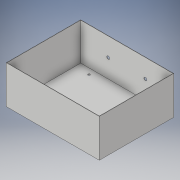
# Autodesk Inventor part: 563-AC-1404-4xSplitter
Saved by Autodesk Inventor 2018 (Build 220112000, 112)
## iProperties
Created: 2018-04-30
Part Number: 563-AC-1404-4xSplitter
Material: Generic
Document SubType Name: Modeling
Designer: bbramman
Density: 1 g/cm^3
Appearance: Default
Author: bbramman
Autodesk Inventor part; units mm, degrees
ref_plane "YZ Plane" through (0, 0, 0) normal (1, 0, 0) x (0, 1, 0)
ref_plane "XZ Plane" through (0, 0, 0) normal (0, 1, 0) x (-1, 0, 0)
ref_plane "XY Plane" through (0, 0, 0) normal (0, 0, 1) x (1, 0, 0)
sketch "Sketch1" plane through (0, 0, 0) normal (0, 1, 0) x (-1, 0, 0)
  line L0 (-63.5, 50.8) -> (63.5, 50.8)
  line L1 (63.5, 50.8) -> (63.5, -50.8)
  line L2 (63.5, -50.8) -> (-63.5, -50.8)
  line L3 (-63.5, -50.8) -> (-63.5, 50.8)
  line L4 (-63.5, 50.8) -> (63.5, -50.8) construction
  line L5 (63.5, 50.8) -> (-63.5, -50.8) construction
  point P0 (0, 0)
  dimension "d0" = 127
  dimension "d1" = 101.6
  constraints: 12 end point, 2 midpoint, 2 parallel, 1 horizontal, 1 perpendicular
  measures "d0" distance of L1.end L2.end
  measures "d1" distance of L0.end L1.end
extrude "Extrusion1" add sketch "Sketch1" along normal blind 1.016
sketch "Sketch2" plane through (0, 1.016, 0) normal (0, 1, 0) x (1, 0, 0)
  line L0 (63.5, 50.8) -> (-63.5, 50.8) projected
  line L1 (63.5, -50.8) -> (-63.5, -50.8)
  line L2 (-63.5, -50.8) -> (-63.5, 50.8)
  line L3 (-63.5, 50.8) -> (63.5, 50.8)
  line L4 (63.5, 50.8) -> (63.5, -50.8)
  line L5 (63.5, -50.8) -> (-63.5, 50.8) construction
  line L6 (-63.5, -50.8) -> (63.5, 50.8) construction
  line L7 (62.992, -50.292) -> (-62.992, -50.292)
  line L8 (-62.992, -50.292) -> (-62.992, 50.292)
  line L9 (-62.992, 50.292) -> (62.992, 50.292)
  line L10 (62.992, 50.292) -> (62.992, -50.292)
  line L11 (62.992, -50.292) -> (-62.992, 50.292) construction
  line L12 (-62.992, -50.292) -> (62.992, 50.292) construction
  point P0 (0, 0)
  dimension "d4" = 125.984
  dimension "d5" = 100.584
  constraints: 24 end point, 4 midpoint, 4 parallel, 2 horizontal, 2 perpendicular
  measures "d4" distance of L8.end L9.end
  measures "d5" distance of L7.end L8.end
extrude "Extrusion2" add sketch "Sketch2" along normal blind 50.8
sketch "Sketch3" plane through (-62.992, 1.016, -50.292) normal (0, 0, 1) x (1, 0, 0)
  line L0 (0, 0) -> (0, 50.8) projected
  circle A0 centre (37.592, 25.4) radius 2.0828
  circle A1 centre (88.392, 25.4) radius 2.0828
  point P0 (62.992, -1.016)
  dimension "d10" = 4.1656
  dimension "d12" = 4.1656
  constraints: 2 centre point
  measures "d10" diameter of A0
  measures "d12" diameter of A1
extrude "Extrusion3" cut sketch "Sketch3" against normal through all
sketch "Sketch4" plane through (0, 1.016, 0) normal (0, 1, 0) x (1, 0, 0)
  line L0 (50, -50) -> (-50, 50) construction
  line L1 (-50, -50) -> (50, 50) construction
  circle A0 centre (-43.65, -42.38) radius 1.4224
  circle A1 centre (-43.65, 42.38) radius 1.4224
  circle A2 centre (41.4402, 7.404) radius 1.4224
  point P0 (0, 0)
  dimension "d15" = 100
  dimension "d16" = 100
  dimension "d23" = 2.8448
  dimension "d24" = 2.8448
  dimension "d25" = 2.8448
  constraints: 4 end point, 3 centre point, 2 midpoint
  measures "d15" distance of L0.end L1.end
  measures "d16" distance of L1.start L0.end
  measures "d23" diameter of A0
  measures "d24" diameter of A1
  measures "d25" diameter of A2
extrude "Extrusion4" cut sketch "Sketch4" against normal through all
body "Solid1"
